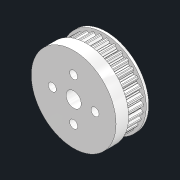
# Autodesk Inventor part: base35
Saved by Autodesk Inventor 2021 (Build 250183000, 183)
## iProperties
Created: 2021-07-14
Part Number: base35
Material: ABS プラスチック
Document SubType Name: Modeling
Designer: yuta0
Density: 1.06 g/cm^3
Appearance: 滑らか - 白
Mass: 10.2844 g
Surface Area: 43.5231 cm^2
Volume: 9.70228 cm^3
Author: yuta0
Autodesk Inventor part; units mm, degrees
ref_plane "YZ Plane" through (0, 0, 0) normal (1, 0, 0) x (0, 1, 0)
ref_plane "XZ Plane" through (0, 0, 0) normal (0, 1, 0) x (-1, 0, 0)
ref_plane "XY Plane" through (0, 0, 0) normal (0, 0, 1) x (1, 0, 0)
sketch "スケッチ1" plane through (0, 0, 0) normal (0, 0, 1) x (1, 0, 0)
  circle A0 centre (0, 0) radius 16.2338 construction
  circle A1 centre (0, 0) radius 15.8528
  circle A2 centre (0, 0) radius 14.7428
  line L0 (-0.975, 16.2045) -> (0.975, 16.2045) construction
  line L1 (-22.7273, 0) -> (22.7273, 0) projected
  circle A3 centre (0.975, 16.2045) radius 1.975
  circle A4 centre (-0.975, 16.2045) radius 1.975
  point P0 (0, 15.8528)
  point P1 (0.3486, 14.7387)
  point P2 (0.9629, 15.8235)
  point P3 (-0.9629, 15.8235)
  point P4 (-0.3486, 14.7387)
  point P5 (0, 15.8528)
  dimension "d1" = 32.4676
  dimension "d2" = 0.381
  dimension "d3" = 1.11
  dimension "d5" = 3.95
  dimension "d6" = 1.95
  dimension "d7" = 3.95
  constraints: 4 centre point, 4 coincident, 2 end point, 2 point on circle, 1 parallel, 1 vertical alignment, 3 other
  measures "d1" diameter of A0
  measures "d5" diameter of A3
  measures "d6" distance of L0.start L0.end
  measures "d7" diameter of A4
extrude "押し出し1" add sketch "スケッチ1" against normal mid plane 7 contours L1 A2 A3 A1 | A1 L1 A2 | A3 A2 A4 A1 | A1 A4 A2 L1 | L1 A2 A4 A3 | A2 L1 | A4 A2 A3 A1 | A3 A4 A2 | A1 A3 A2 A4 | A4 A3 A2 | A4 A2 A3
extrude "押し出し2" cut sketch "スケッチ1" against normal through all both and the other way through all contours A4 A2 A3 A1 picked at (0.0387, 15.4805)
fillet "フィレット1" radius 0.285 2 edges at (0.9629, 15.8235, 0) (-0.9629, 15.8235, 0)
fillet "フィレット2" radius 0.15 2 edges at (0.3486, 14.7387, 0) (-0.3486, 14.7387, 0)
pattern_circular "円形状パターン1" count 34 over 360 about axis through (0, 0, -10) along (0, 0, 1) of "押し出し2", "フィレット1", "フィレット2"
sketch "スケッチ9" plane through (0, 0, -3.5) normal (0, 0, -1) x (-1, 0, 0)
  circle A0 centre (0, 0) radius 16.8528
  arc A1 (-1.2014, 15.8072) -> (-1.7236, 15.7588) centre (0, 0) ccw projected
  dimension "d59" = 1
  constraints: 1 centre point, 1 coincident
  measures "d59" radial gap between concentric circles of A0 A1
extrude "押し出し8" add sketch "スケッチ9" along normal blind 1
mirror "ミラー1" about plane through (0, 0, 0) normal (0, 0, 1) of "押し出し8"
sketch "スケッチ11" plane through (0, 0, 4.5) normal (0, 0, 1) x (1, 0, 0)
  circle A0 centre (0, 0) radius 16.8528
  circle A1 centre (0, 0) radius 16.8528 projected
  dimension "d66" = 0
  constraints: 1 centre point, 1 coincident
  measures "d66" radial gap between concentric circles of A1 A0
extrude "押し出し10" add sketch "スケッチ11" along normal blind 4
sketch "スケッチ2" plane through (0, 0, -4.5) normal (0, 0, -1) x (1, 0, 0)
  circle A0 centre (0, 0) radius 8.5
  point P0 (0, 8.5)
  point P1 (-8.5, 0)
  point P2 (0, -8.5)
  point P3 (8.5, 0)
  dimension "d17" = 17
  dimension "d20" = 360
  constraints: 1 coincident, 1 vertical alignment, 7 other
hole "穴1" at (8.5, 0, -4.5) at (0, 8.5, -4.5) at (-8.5, 0, -4.5) at (0, -8.5, -4.5) direction (0, 0, 1) diameter 3.2 end through all counterbore diameter 6.5 counterbore depth 3 clearance for "Socket Head Cap Screw" size "M3" standard "Ansi Metric M Profile"
sketch "スケッチ10" plane through (0, 0, -4.5) normal (0, 0, -1) x (-1, 0, 0)
  circle A0 centre (0, 0) radius 3
  dimension "d60" = 6
  constraints: 1 centre point, 1 coincident
  measures "d60" diameter of A0
extrude "押し出し9" cut sketch "スケッチ10" against normal through all
equation "\"d7\" = d5"
